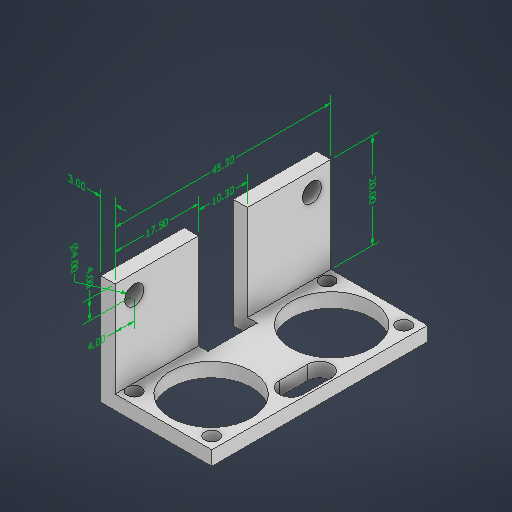
# Autodesk Inventor part: USSensorBracket
Saved by Autodesk Inventor 2026 (Build 300175000, 175)
## iProperties
Created: 2025-07-21
Part Number: USSensorBracket
Material: Generic
Document SubType Name: Modeling
Designer: jsmal
Density: 1 g/cm^3
Appearance: Default
Author: jsmal
Autodesk Inventor part; units mm, degrees
ref_plane "YZ Plane" through (0, 0, 0) normal (1, 0, 0) x (0, 1, 0)
ref_plane "XZ Plane" through (0, 0, 0) normal (0, 1, 0) x (-1, 0, 0)
ref_plane "XY Plane" through (0, 0, 0) normal (0, 0, 1) x (1, 0, 0)
sketch "Sketch1" plane through (0, 0, 0) normal (0, 1, 0) x (-1, 0, 0)
  line L0 (0, 0) -> (20.3, 0)
  line L1 (20.3, 0) -> (20.3, -45.3)
  line L2 (20.3, -45.3) -> (0, -45.3)
  line L3 (0, -45.3) -> (0, 0)
  dimension "d0" = 20.3
  dimension "d1" = 45.3
  constraints: 8 end point, 2 parallel, 1 horizontal, 1 perpendicular
  measures "d0" distance of L1.end L2.end
  measures "d1" distance of L0.end L1.end
extrude "Extrusion1" add sketch "Sketch1" along normal blind 3
sketch "Sketch2" plane through (0, 3, 0) normal (0, 1, 0) x (1, 0, 0)
  circle A0 centre (-10.15, 10) radius 8.5
  line L0 (-20.3, 45.3) -> (-20.3, 0) projected
  line L1 (0, 0) -> (0, 45.3) projected
  line L2 (-20.3, 0) -> (0, 0) projected
  circle A1 centre (-10.15, 35.3) radius 8.5
  line L3 (0, 45.3) -> (-20.3, 45.3) projected
  dimension "d4" = 17
  dimension "d5" = 10.15
  dimension "d6" = 10.15
  dimension "d7" = 10
  dimension "d8" = 17
  dimension "d9" = 10.15
  dimension "d10" = 10
  constraints: 2 centre point
  measures "d4" diameter of A0
  measures "d5" distance from line of L0 A0.centre
  measures "d6" distance from line of L1 A0.centre
  measures "d7" distance from line of L2 A0.centre
  measures "d8" diameter of A1
  measures "d9" distance from line of L0 A1.centre
  measures "d10" distance from line of L3 A1.centre
extrude "Extrusion2" cut sketch "Sketch2" against normal blind 3 contours A0 | A1
sketch "Sketch3" plane through (-20.3, 0, -45.3) normal (-1, 0, 0) x (0, 0, 1)
  line L0 (45.3, 3) -> (0, 3) projected
  line L1 (45.3, 0) -> (27.8, 0)
  line L2 (27.8, 0) -> (27.8, 3)
  line L3 (27.8, 3) -> (45.3, 3)
  line L4 (45.3, 3) -> (45.3, 0)
  line L5 (0, 0) -> (17.5, 0)
  line L6 (17.5, 0) -> (17.5, 3)
  line L7 (17.5, 3) -> (0, 3)
  line L8 (0, 3) -> (0, 0)
  point P0 (0, 3)
  dimension "d13" = 17.5
  dimension "d14" = 17.5
  constraints: 16 end point, 4 parallel, 3 point on line, 2 horizontal, 2 perpendicular
  measures "d13" distance of L2.end L3.end
  measures "d14" distance of L7.end L6.end
extrude "Extrusion3" add sketch "Sketch3" along normal blind 3
sketch "Sketch4" plane through (0, 3, 0) normal (0, 1, 0) x (1, 0, 0)
  line L0 (0, 0) -> (-23.3, 0) projected
  line L1 (0, 45.3) -> (-23.3, 45.3) projected
  line L2 (-23.3, 0) -> (-20.3, 0)
  line L3 (-20.3, 0) -> (-20.3, 45.3)
  line L4 (-20.3, 45.3) -> (-23.3, 45.3)
  line L5 (-23.3, 45.3) -> (-23.3, 0)
  dimension "d17" = 3
  constraints: 8 end point, 2 parallel, 1 horizontal, 1 perpendicular, 1 point on line
  measures "d17" distance of L4.end L3.end
extrude "Extrusion4" add sketch "Sketch4" along normal blind 20
sketch "Sketch5" plane through (-23.3, 0, -45.3) normal (-1, 0, 0) x (0, 0, 1)
  line L0 (27.8, 0) -> (27.8, 3) projected
  line L1 (27.8, 3) -> (17.5, 3)
  line L2 (17.5, 3) -> (17.5, 23)
  line L3 (17.5, 23) -> (27.8, 23)
  line L4 (27.8, 23) -> (27.8, 3)
  line L5 (17.5, 0) -> (17.5, 3) projected
  point P0 (45.3, 0)
  dimension "d20" = 10.3
  dimension "d21" = 0
  dimension "d22" = 20
  constraints: 8 end point, 2 parallel, 1 horizontal, 1 perpendicular
  measures "d20" distance of L2.end L3.end
  measures "d21" distance between parallel lines of L5 L2
  measures "d22" distance of L3.end L0.end
extrude "Extrusion5" cut sketch "Sketch5" against normal blind 3
sketch "Sketch6" plane through (0, 0, 0) normal (0, -1, 0) x (1, 0, 0)
  line L0 (-3, -28.15) -> (-3, -17.15) construction
  line L1 (-0.5, -25.65) -> (-0.5, -19.65)
  line L2 (-5.5, -19.65) -> (-5.5, -25.65)
  arc A0 (-5.5, -25.65) -> (-0.5, -25.65) centre (-3, -25.65) ccw
  arc A1 (-0.5, -19.65) -> (-5.5, -19.65) centre (-3, -19.65) ccw
  line L3 (0, 0) -> (0, -45.3) projected
  line L4 (0, -45.3) -> (-23.3, -45.3) projected
  point P0 (-3, -22.65)
  dimension "d25" = 11
  dimension "d26" = 5
  dimension "d27" = 0.5
  dimension "d28" = 22.65
  constraints: 8 end point, 6 point on circle, 4 tangent, 2 centre point, 2 point on line, 1 midpoint, 1 parallel, 1 vertical
  measures "d25" distance of L0.start L0.end
  measures "d26" diameter of A1
  measures "d27" distance between parallel lines of L3 L1
  measures "d28" distance from line of L4 point (-3, -22.65)
extrude "Extrusion6" cut sketch "Sketch6" against normal blind 3
sketch "Sketch7" plane through (0, 0, 0) normal (0, -1, 0) x (1, 0, 0)
  line L0 (-20.3, -27.8) -> (-20.3, -17.5) projected
  line L1 (-20.3, -27.8) -> (-18.3, -27.8)
  line L2 (-18.3, -27.8) -> (-18.3, -17.5)
  line L3 (-18.3, -17.5) -> (-20.3, -17.5)
  line L4 (-20.3, -17.5) -> (-20.3, -27.8)
  point P0 (0, 0)
  dimension "d31" = 2
  constraints: 8 end point, 2 parallel, 1 horizontal, 1 perpendicular
  measures "d31" distance of L3.end L2.end
extrude "Extrusion7" cut sketch "Sketch7" against normal blind 3
sketch "Sketch8" plane through (0, 0, 0) normal (0, -1, 0) x (1, 0, 0)
  line L0 (0, 0) -> (0, -45.3) projected
  line L1 (0, -45.3) -> (-23.3, -45.3) projected
  line L2 (0, 0) -> (-23.3, 0) projected
  point P0 (-2.5, -2.5)
  point P1 (-18.8095, -2.5)
  point P2 (-18.6137, -42.8)
  point P3 (-2.5, -42.8)
  dimension "d52" = 2.5
  dimension "d53" = 2.5
  dimension "d54" = 2.5
  dimension "d55" = 2.5
  dimension "d56" = 2.5
  dimension "d57" = 2.5
  measures "d52" distance from line of L0 point (-2.5, -42.8)
  measures "d53" distance from line of L1 point (-2.5, -42.8)
  measures "d54" distance from line of L0 point (-2.5, -2.5)
  measures "d55" distance from line of L2 point (-2.5, -2.5)
  measures "d56" distance from line of L2 point (-18.809, -2.5)
  measures "d57" distance from line of L1 point (-18.614, -42.8)
hole "Hole1" at (-2.5, 0, -42.8) at (-2.5, 0, -2.5) at (-18.8095, 0, -2.5) at (-18.6137, 0, -42.8) direction (0, 1, 0) diameter 3 depth 3 tip angle 118
sketch "Sketch9" plane through (-23.3, 0, -45.3) normal (-1, 0, 0) x (0, 0, 1)
  line L0 (0, 23) -> (45.3, 23) projected
  line L1 (0, 0) -> (0, 23) projected
  line L2 (45.3, 0) -> (45.3, 23) projected
  point P0 (4, 19)
  point P1 (41.3, 19)
  dimension "d41" = 4
  dimension "d49" = 4
  dimension "d50" = 4
  dimension "d51" = 4
  measures "d41" distance from line of L0 point (4, 19)
  measures "d49" distance from line of L1 point (4, 19)
  measures "d50" distance from line of L0 point (41.3, 19)
  measures "d51" distance from line of L2 point (41.3, 19)
hole "Hole2" at (-23.3, 19, -41.3) at (-23.3, 19, -4) direction (1, 0, 0) diameter 4 depth 3 tip angle 118
body "Solid1"
